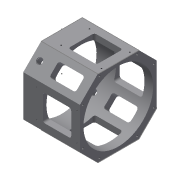
# Autodesk Inventor part: Chamber_wall_NEW_v_4
Saved by Autodesk Inventor 2013 (Build 170138000, 138)
## iProperties
Created: 2012-06-12
Part Number: Chamber_wall_NEW_v_4
Material: Generic
Document SubType Name: Sheet Metal
Designer: Breckenridge2 User
Density: 1 g/cm^3
Sheet Metal Rule: Default
Author: Breckenridge2 User
Autodesk Inventor part; units mm, degrees
ref_plane "YZ Plane" through (0, 0, 0) normal (1, 0, 0) x (0, 1, 0)
ref_plane "XZ Plane" through (0, 0, 0) normal (0, 1, 0) x (-1, 0, 0)
ref_plane "XY Plane" through (0, 0, 0) normal (0, 0, 1) x (1, 0, 0)
sketch "Sketch1" plane through (0, 0, 0) normal (1, 0, 0) x (0, 1, 0)
  point P0 (0, 0)
sketch "Sketch2" plane through (0, 0, 0) normal (1, 0, 0) x (0, 1, 0)
  circle A0 centre (0, 0) radius 101.6
  line L0 (-59.69, 112.014) -> (59.69, 112.014)
  line L1 (59.69, -112.014) -> (-59.69, -112.014)
  line L2 (-59.69, 112.014) -> (59.69, -112.014) construction
  line L3 (59.69, 112.014) -> (-59.69, -112.014) construction
  line L4 (112.014, 59.69) -> (112.014, -59.69)
  line L5 (-112.014, -59.69) -> (-112.014, 59.69)
  line L6 (-112.014, 59.69) -> (112.014, -59.69) construction
  line L7 (112.014, 59.69) -> (-112.014, -59.69) construction
  line L8 (-112.014, 59.69) -> (-59.69, 112.014)
  line L9 (59.69, 112.014) -> (112.014, 59.69)
  line L10 (112.014, -59.69) -> (59.69, -112.014)
  line L11 (-59.69, -112.014) -> (-112.014, -59.69)
  dimension "d1" = 203.2
  dimension "d2" = 119.38
  dimension "d3" = 224.028
  dimension "d4" = 224.028
  dimension "d5" = 119.38
  constraints: 24 end point, 4 midpoint, 2 parallel, 1 centre point, 1 horizontal
  measures "d1" diameter of A0
  measures "d2" distance of L1.start L1.end
  measures "d3" distance of L0.end L1.start
  measures "d4" distance of L4.end L5.start
  measures "d5" distance of L4.start L4.end
extrude "Extrusion1" add sketch "Sketch2" along normal blind 165.1
sketch "Sketch3" plane through (0, 112.014, 59.69) normal (0, 1, 0) x (1, 0, 0)
  line L0 (0, 0) -> (0, 119.38) projected
  line L1 (0, 0) -> (165.1, 0) projected
  line L2 (165.1, 119.38) -> (165.1, 0) projected
  line L3 (0, 119.38) -> (165.1, 119.38) projected
  point P0 (0, 59.69)
sketch "Sketch4" plane through (0, 112.014, 59.69) normal (0, 1, 0) x (1, 0, 0)
  line L0 (133.35, 97.79) -> (63.5, 97.79)
  line L1 (57.15, 91.44) -> (57.15, 27.94)
  line L2 (63.5, 21.59) -> (133.35, 21.59)
  line L3 (139.7, 27.94) -> (139.7, 91.44)
  arc A0 (63.5, 97.79) -> (57.15, 91.44) centre (63.5, 91.44) ccw
  arc A1 (139.7, 91.44) -> (133.35, 97.79) centre (133.35, 91.44) ccw
  arc A2 (133.35, 21.59) -> (139.7, 27.94) centre (133.35, 27.94) ccw
  arc A3 (57.15, 27.94) -> (63.5, 21.59) centre (63.5, 27.94) ccw
  point P0 (0, 59.69)
  point P1 (57.15, 21.59)
  point P2 (57.15, 97.79)
  point P3 (139.7, 21.59)
  dimension "d10" = 82.55
  dimension "d11" = 76.2
  dimension "d12" = 6.35
  constraints: 8 end point, 8 point on circle, 8 tangent, 6 point on line, 4 centre point, 3 equal radius, 2 parallel, 1 horizontal, 1 perpendicular
  measures "d10" distance of point (139.7, 21.59) point (57.15, 21.59)
  measures "d11" distance of point (57.15, 21.59) point (57.15, 97.79)
  measures "d12" radius of A0
extrude "Cut1" cut sketch "Sketch4" against normal up to next
sketch "Sketch5" plane through (0, 112.014, 59.69) normal (0, 1, 0) x (1, 0, 0)
  line L0 (0, 0) -> (0, 119.38) projected
  line L1 (0, 0) -> (165.1, 0) projected
  line L2 (165.1, 119.38) -> (165.1, 0) projected
  line L3 (0, 119.38) -> (165.1, 119.38) projected
  point P0 (0, 59.69)
sketch "Sketch6" plane through (0, -59.69, -112.014) normal (0, 0, -1) x (-1, 0, 0)
  line L0 (-133.35, 97.79) -> (-63.5, 97.79)
  line L1 (-57.15, 91.44) -> (-57.15, 27.94)
  line L2 (-63.5, 21.59) -> (-133.35, 21.59)
  line L3 (-139.7, 27.94) -> (-139.7, 91.44)
  arc A0 (-57.15, 91.44) -> (-63.5, 97.79) centre (-63.5, 91.44) ccw
  arc A1 (-63.5, 21.59) -> (-57.15, 27.94) centre (-63.5, 27.94) ccw
  arc A2 (-133.35, 97.79) -> (-139.7, 91.44) centre (-133.35, 91.44) ccw
  arc A3 (-139.7, 27.94) -> (-133.35, 21.59) centre (-133.35, 27.94) ccw
  point P0 (0, 59.69)
  point P1 (-57.15, 21.59)
  point P2 (-57.15, 97.79)
  point P3 (-139.7, 21.59)
  dimension "d17" = 82.55
  dimension "d18" = 76.2
  dimension "d19" = 6.35
  constraints: 8 end point, 8 point on circle, 8 tangent, 6 point on line, 4 centre point, 3 equal radius, 2 parallel, 1 horizontal, 1 perpendicular
  measures "d17" distance of point (-57.15, 21.59) point (-139.7, 21.59)
  measures "d18" distance of point (-57.15, 97.79) point (-57.15, 21.59)
  measures "d19" radius of A0
extrude "Cut2" cut sketch "Sketch6" against normal up to next
sketch "Sketch7" plane through (0, -112.014, -59.69) normal (0, -1, 0) x (1, 0, 0)
  line L0 (0, 0) -> (0, 119.38) projected
  line L1 (0, 0) -> (165.1, 0) projected
  line L2 (165.1, 119.38) -> (165.1, 0) projected
  line L3 (0, 119.38) -> (165.1, 119.38) projected
  point P0 (0, 59.69)
sketch "Sketch8" plane through (165.1, -59.69, -112.014) normal (0, -0.7071068, -0.7071068) x (-1, 0, 0)
  line L0 (165.1, 0) -> (165.1, -73.9973) projected
  line L1 (165.1, 0) -> (0, 0) projected
  line L2 (0, -73.9973) -> (0, 0) projected
  line L3 (165.1, -73.9973) -> (0, -73.9973) projected
  point P0 (165.1, -36.9987)
sketch "Sketch9" plane through (0, -112.014, -59.69) normal (0, -1, 0) x (1, 0, 0)
  line L0 (133.35, 97.79) -> (63.5, 97.79)
  line L1 (57.15, 91.44) -> (57.15, 27.94)
  line L2 (63.5, 21.59) -> (133.35, 21.59)
  line L3 (139.7, 27.94) -> (139.7, 91.44)
  arc A0 (63.5, 97.79) -> (57.15, 91.44) centre (63.5, 91.44) ccw
  arc A1 (139.7, 91.44) -> (133.35, 97.79) centre (133.35, 91.44) ccw
  arc A2 (133.35, 21.59) -> (139.7, 27.94) centre (133.35, 27.94) ccw
  arc A3 (57.15, 27.94) -> (63.5, 21.59) centre (63.5, 27.94) ccw
  point P0 (0, 59.69)
  point P1 (57.15, 21.59)
  point P2 (57.15, 97.79)
  point P3 (139.7, 21.59)
  dimension "d24" = 82.55
  dimension "d25" = 76.2
  dimension "d26" = 6.35
  constraints: 8 end point, 8 point on circle, 8 tangent, 6 point on line, 4 centre point, 3 equal radius, 2 parallel, 1 horizontal, 1 perpendicular
  measures "d24" distance of point (139.7, 21.59) point (57.15, 21.59)
  measures "d25" distance of point (57.15, 21.59) point (57.15, 97.79)
  measures "d26" radius of A0
extrude "Cut3" cut sketch "Sketch9" against normal up to next
sketch "Sketch10" plane through (0, -59.69, 112.014) normal (0, 0, 1) x (1, 0, 0)
  line L0 (133.35, 97.79) -> (63.5, 97.79)
  line L1 (57.15, 91.44) -> (57.15, 27.94)
  line L2 (63.5, 21.59) -> (133.35, 21.59)
  line L3 (139.7, 27.94) -> (139.7, 91.44)
  arc A0 (63.5, 97.79) -> (57.15, 91.44) centre (63.5, 91.44) ccw
  arc A1 (57.15, 27.94) -> (63.5, 21.59) centre (63.5, 27.94) ccw
  arc A2 (139.7, 91.44) -> (133.35, 97.79) centre (133.35, 91.44) ccw
  arc A3 (133.35, 21.59) -> (139.7, 27.94) centre (133.35, 27.94) ccw
  point P0 (57.15, 21.59)
  point P1 (57.15, 97.79)
  point P2 (139.7, 21.59)
  dimension "d31" = 82.55
  dimension "d32" = 76.2
  constraints: 8 end point, 8 point on circle, 8 tangent, 6 point on line, 4 centre point, 3 equal radius, 2 parallel, 1 horizontal, 1 perpendicular
  measures "d31" distance of point (139.7, 21.59) point (57.15, 21.59)
  measures "d32" distance of point (57.15, 21.59) point (57.15, 97.79)
extrude "Cut4" cut sketch "Sketch10" against normal up to next
sketch "Sketch11" plane through (165.1, -59.69, -112.014) normal (0, -0.7071068, -0.7071068) x (-1, 0, 0)
  line L0 (0, 0) -> (25.4, 0)
  line L1 (25.4, 0) -> (25.4, -17.907)
  line L2 (31.75, -17.907) -> (95.25, -17.907)
  line L3 (101.6, -24.257) -> (101.6, -49.657)
  line L4 (95.25, -56.007) -> (31.75, -56.007)
  line L5 (25.4, -49.657) -> (25.4, -24.257)
  arc A0 (101.6, -24.257) -> (95.25, -17.907) centre (95.25, -24.257) ccw
  arc A1 (95.25, -56.007) -> (101.6, -49.657) centre (95.25, -49.657) ccw
  arc A2 (25.4, -49.657) -> (31.75, -56.007) centre (31.75, -49.657) ccw
  arc A3 (31.75, -17.907) -> (25.4, -24.257) centre (31.75, -24.257) ccw
  point P0 (165.1, -36.9987)
  point P1 (101.6, -56.007)
  point P2 (101.6, -17.907)
  point P3 (25.4, -56.007)
  dimension "d37" = 17.907
  dimension "d38" = 76.2
  dimension "d39" = 38.1
  dimension "d40" = 6.35
  constraints: 12 end point, 8 point on circle, 8 point on line, 8 tangent, 4 centre point, 3 equal radius, 2 horizontal, 2 parallel, 2 perpendicular
  measures "d37" distance of L0.end L1.end
  measures "d38" distance of point (101.6, -56.007) point (25.4, -56.007)
  measures "d39" distance of point (101.6, -17.907) point (101.6, -56.007)
  measures "d40" radius of A0
extrude "Cut5" cut sketch "Sketch11" against normal up to next
sketch "Sketch12" plane through (165.1, -59.69, -112.014) normal (0, -0.7071068, -0.7071068) x (-1, 0, 0)
  line L0 (0, 0) -> (143.51, 0)
  line L1 (143.51, 0) -> (143.51, -36.957)
  line L2 (143.51, -36.957) -> (0, -36.957)
  line L3 (0, -36.957) -> (0, 0)
  circle A0 centre (143.51, -36.957) radius 7.9375
  circle A1 centre (143.51, -36.957) radius 8.6995
  point P0 (165.1, -36.9987)
  dimension "d43" = 143.51
  dimension "d44" = 36.957
  dimension "d45" = 15.875
  dimension "d46" = 17.399
  constraints: 8 end point, 2 centre point, 2 coincident, 2 parallel, 1 horizontal, 1 perpendicular
  measures "d43" distance of L1.end L2.end
  measures "d44" distance of L0.end L1.end
  measures "d45" diameter of A0
  measures "d46" diameter of A1
extrude "Cut6" cut sketch "Sketch12" against normal up to next contours A0 L2 L1 | L1 L2 A0
sketch "Sketch13" plane through (165.1, -59.69, -112.014) normal (0, -0.7071068, -0.7071068) x (-1, 0, 0)
  circle A0 centre (143.51, -36.957) radius 7.9375 projected
  circle A1 centre (143.51, -36.957) radius 8.6995
  point P0 (165.1, -36.9987)
  dimension "d49" = 17.399
  constraints: 1 centre point, 1 coincident
  measures "d49" diameter of A1
extrude "Cut7" cut sketch "Sketch13" against normal blind 2.54
sketch "Sketch14" plane through (165.1, 112.014, -59.69) normal (0, 0.7071068, -0.7071068) x (-1, 0, 0)
  line L0 (31.75, -17.907) -> (95.25, -17.907)
  line L1 (101.6, -24.257) -> (101.6, -49.657)
  line L2 (95.25, -56.007) -> (31.75, -56.007)
  line L3 (25.4, -49.657) -> (25.4, -24.257)
  arc A0 (101.6, -24.257) -> (95.25, -17.907) centre (95.25, -24.257) ccw
  arc A1 (95.25, -56.007) -> (101.6, -49.657) centre (95.25, -49.657) ccw
  arc A2 (25.4, -49.657) -> (31.75, -56.007) centre (31.75, -49.657) ccw
  arc A3 (31.75, -17.907) -> (25.4, -24.257) centre (31.75, -24.257) ccw
  point P0 (165.1, -36.9987)
  point P1 (101.6, -56.007)
  point P2 (101.6, -17.907)
  point P3 (25.4, -56.007)
  dimension "d54" = 76.2
  dimension "d55" = 38.1
  dimension "d56" = 6.35
  constraints: 8 end point, 8 point on circle, 8 tangent, 6 point on line, 4 centre point, 3 equal radius, 2 parallel, 1 horizontal, 1 perpendicular
  measures "d54" distance of point (101.6, -56.007) point (25.4, -56.007)
  measures "d55" distance of point (101.6, -17.907) point (101.6, -56.007)
  measures "d56" radius of A0
extrude "Cut8" cut sketch "Sketch14" against normal up to next
sketch "Sketch15" plane through (165.1, 112.014, -59.69) normal (0, 0.7071068, -0.7071068) x (-1, 0, 0)
  line L0 (0, 0) -> (143.51, 0)
  line L1 (143.51, 0) -> (143.51, -36.957)
  line L2 (143.51, -36.957) -> (0, -36.957)
  line L3 (0, -36.957) -> (0, 0)
  circle A0 centre (143.51, -36.957) radius 7.9375
  point P0 (165.1, -36.9987)
  dimension "d59" = 143.51
  dimension "d60" = 36.957
  dimension "d61" = 15.875
  constraints: 8 end point, 2 parallel, 1 centre point, 1 coincident, 1 horizontal, 1 perpendicular
  measures "d59" distance of L1.end L2.end
  measures "d60" distance of L0.end L1.end
  measures "d61" diameter of A0
extrude "Cut9" cut sketch "Sketch15" against normal up to next contours A0 L2 L1 | L1 L2 A0
sketch "Sketch16" plane through (165.1, 112.014, -59.69) normal (0, 0.7071068, -0.7071068) x (-1, 0, 0)
  circle A0 centre (143.51, -36.957) radius 7.9375 projected
  circle A1 centre (143.51, -36.957) radius 8.6995
  point P0 (165.1, -36.9987)
  dimension "d64" = 17.399
  constraints: 1 centre point, 1 coincident
  measures "d64" diameter of A1
extrude "Cut10" cut sketch "Sketch16" against normal blind 2.54
sketch "Sketch17" plane through (0, 59.69, 112.014) normal (0, 0.7071068, 0.7071068) x (1, 0, 0)
  line L0 (133.35, 56.0903) -> (69.85, 56.0903)
  line L1 (63.5, 49.7403) -> (63.5, 24.3403)
  line L2 (69.85, 17.9903) -> (133.35, 17.9903)
  line L3 (139.7, 24.3403) -> (139.7, 49.7403)
  arc A0 (69.85, 56.0903) -> (63.5, 49.7403) centre (69.85, 49.7403) ccw
  arc A1 (139.7, 49.7403) -> (133.35, 56.0903) centre (133.35, 49.7403) ccw
  arc A2 (133.35, 17.9903) -> (139.7, 24.3403) centre (133.35, 24.3403) ccw
  arc A3 (63.5, 24.3403) -> (69.85, 17.9903) centre (69.85, 24.3403) ccw
  point P0 (0, 36.9987)
  point P1 (63.5, 17.9903)
  point P2 (63.5, 56.0903)
  point P3 (139.7, 17.9903)
  dimension "d69" = 76.2
  dimension "d70" = 38.1
  dimension "d71" = 6.35
  constraints: 8 end point, 8 point on circle, 8 tangent, 6 point on line, 4 centre point, 3 equal radius, 2 parallel, 1 horizontal, 1 perpendicular
  measures "d69" distance of point (139.7, 17.99) point (63.5, 17.99)
  measures "d70" distance of point (63.5, 17.99) point (63.5, 56.09)
  measures "d71" radius of A0
extrude "Cut11" cut sketch "Sketch17" against normal up to next
sketch "Sketch18" plane through (0, 59.69, 112.014) normal (0, 0.7071068, 0.7071068) x (1, 0, 0)
  line L0 (165.1, 0) -> (21.59, 0)
  line L1 (21.59, 0) -> (21.59, 36.957)
  line L2 (21.59, 36.957) -> (165.1, 36.957)
  line L3 (165.1, 36.957) -> (165.1, 0)
  circle A0 centre (21.59, 36.957) radius 7.9375
  point P0 (0, 36.9987)
  dimension "d74" = 143.51
  dimension "d75" = 36.957
  dimension "d76" = 15.875
  constraints: 8 end point, 2 parallel, 1 centre point, 1 coincident, 1 horizontal, 1 perpendicular
  measures "d74" distance of L1.end L2.end
  measures "d75" distance of L0.end L1.end
  measures "d76" diameter of A0
extrude "Cut12" cut sketch "Sketch18" against normal up to next contours A0 L2 L1 | L1 L2 A0
sketch "Sketch19" plane through (0, 59.69, 112.014) normal (0, 0.7071068, 0.7071068) x (1, 0, 0)
  circle A0 centre (21.59, 36.957) radius 7.9375 projected
  circle A1 centre (21.59, 36.957) radius 8.6995
  point P0 (0, 36.9987)
  dimension "d79" = 17.399
  constraints: 1 centre point, 1 coincident
  measures "d79" diameter of A1
extrude "Cut13" cut sketch "Sketch19" against normal blind 2.54
sketch "Sketch20" plane through (0, -112.014, 59.69) normal (0, -0.7071068, 0.7071068) x (1, 0, 0)
  line L0 (133.35, 56.0903) -> (69.85, 56.0903)
  line L1 (63.5, 49.7403) -> (63.5, 24.3403)
  line L2 (69.85, 17.9903) -> (133.35, 17.9903)
  line L3 (139.7, 24.3403) -> (139.7, 49.7403)
  arc A0 (69.85, 56.0903) -> (63.5, 49.7403) centre (69.85, 49.7403) ccw
  arc A1 (139.7, 49.7403) -> (133.35, 56.0903) centre (133.35, 49.7403) ccw
  arc A2 (133.35, 17.9903) -> (139.7, 24.3403) centre (133.35, 24.3403) ccw
  arc A3 (63.5, 24.3403) -> (69.85, 17.9903) centre (69.85, 24.3403) ccw
  point P0 (0, 36.9987)
  point P1 (63.5, 17.9903)
  point P2 (63.5, 56.0903)
  point P3 (139.7, 17.9903)
  dimension "d84" = 76.2
  dimension "d85" = 38.1
  dimension "d86" = 6.35
  constraints: 8 end point, 8 point on circle, 8 tangent, 6 point on line, 4 centre point, 3 equal radius, 2 parallel, 1 horizontal, 1 perpendicular
  measures "d84" distance of point (139.7, 17.99) point (63.5, 17.99)
  measures "d85" distance of point (63.5, 17.99) point (63.5, 56.09)
  measures "d86" radius of A0
extrude "Cut14" cut sketch "Sketch20" against normal up to next
sketch "Sketch21" plane through (0, -112.014, 59.69) normal (0, -0.7071068, 0.7071068) x (1, 0, 0)
  line L0 (165.1, 0) -> (21.59, 0)
  line L1 (21.59, 0) -> (21.59, 36.957)
  line L2 (21.59, 36.957) -> (165.1, 36.957)
  line L3 (165.1, 36.957) -> (165.1, 0)
  circle A0 centre (21.59, 36.957) radius 7.9375
  point P0 (0, 36.9987)
  dimension "d89" = 143.51
  dimension "d90" = 36.957
  dimension "d91" = 15.875
  constraints: 8 end point, 2 parallel, 1 centre point, 1 coincident, 1 horizontal, 1 perpendicular
  measures "d89" distance of L1.end L2.end
  measures "d90" distance of L0.end L1.end
  measures "d91" diameter of A0
extrude "Cut15" cut sketch "Sketch21" against normal up to next contours A0 L2 L1 | L1 L2 A0
sketch "Sketch22" plane through (0, -112.014, 59.69) normal (0, -0.7071068, 0.7071068) x (1, 0, 0)
  circle A0 centre (21.59, 36.957) radius 7.9375 projected
  circle A1 centre (21.59, 36.957) radius 8.6995
  point P0 (0, 36.9987)
  dimension "d94" = 17.399
  constraints: 1 centre point, 1 coincident
  measures "d94" diameter of A1
extrude "Cut16" cut sketch "Sketch22" against normal blind 2.54
sketch "Sketch23" plane through (165.1, 0, 0) normal (1, 0, 0) x (0, 0, -1)
  point P0 (-103.1134, 54.9471)
  point P1 (-54.9471, 103.1134)
  point P2 (54.9471, 103.1134)
  point P3 (103.1134, 54.9471)
  point P4 (103.1134, -54.9471)
  point P5 (54.9471, -103.1134)
  point P6 (-54.9471, -103.1134)
  point P7 (-103.1134, -54.9471)
hole "Hole1" at (165.1, 54.9471, 103.1134) at (165.1, 103.1134, 54.9471) at (165.1, 103.1134, -54.9471) at (165.1, 54.9471, -103.1134) at (165.1, -54.9471, -103.1134) at (165.1, -103.1134, -54.9471) at (165.1, -103.1134, 54.9471) at (165.1, -54.9471, 103.1134) direction (-1, 0, 0) diameter 4.9784 depth 18.415 tip angle 118 thread size "1/4-20 UNC" class "2B" standard "ANSI Unified Screw Threads"
sketch "Sketch24" plane through (0, 0, 0) normal (-1, 0, 0) x (0, 0, 1)
  point P0 (-103.1134, 54.9471)
  point P1 (-54.9471, 103.1134)
  point P2 (54.9471, 103.1134)
  point P3 (103.1134, 54.9471)
  point P4 (103.1134, -54.9471)
  point P5 (54.9471, -103.1134)
  point P6 (-54.9471, -103.1134)
  point P7 (-103.1134, -54.9471)
hole "Hole2" at (0, 54.9471, -103.1134) at (0, 103.1134, -54.9471) at (0, 103.1134, 54.9471) at (0, 54.9471, 103.1134) at (0, -54.9471, 103.1134) at (0, -103.1134, 54.9471) at (0, -103.1134, -54.9471) at (0, -54.9471, -103.1134) direction (1, 0, 0) diameter 4.9784 depth 18.415 tip angle 118 thread size "1/4-20 UNC" class "2B" standard "ANSI Unified Screw Threads"
sketch "Sketch25" plane through (0, -59.69, 112.014) normal (0, 0, 1) x (1, 0, 0)
  point P0 (0, 59.69)
  point P1 (157.226, 100.965)
  point P2 (39.624, 100.965)
  point P3 (39.624, 18.415)
  point P4 (157.226, 18.415)
hole "Hole3" at (39.624, 41.275, 112.014) at (157.226, 41.275, 112.014) at (39.624, -41.275, 112.014) at (157.226, -41.275, 112.014) direction (0, 0, -1) diameter 3.9624 depth 13.97 tip angle 118 thread size "10-32 UNF" class "2B" standard "ANSI Unified Screw Threads"
sketch "Sketch26" plane through (0, 112.014, 59.69) normal (0, 1, 0) x (1, 0, 0)
  point P0 (0, 59.69)
  point P1 (157.226, 100.965)
  point P2 (39.624, 100.965)
  point P3 (39.624, 18.415)
  point P4 (157.226, 18.415)
  point P5 (157.226, 100.965)
  constraints: 1 coincident
hole "Hole4" at (39.624, 112.014, 41.275) at (39.624, 112.014, -41.275) at (157.226, 112.014, -41.275) at (157.226, 112.014, 41.275) direction (0, -1, 0) diameter 3.9624 depth 13.97 tip angle 118 thread size "10-32 UNF" class "2B" standard "ANSI Unified Screw Threads"
sketch "Sketch27" plane through (0, -112.014, -59.69) normal (0, -1, 0) x (1, 0, 0)
  point P0 (0, 59.69)
  point P1 (157.226, 100.965)
  point P2 (39.624, 100.965)
  point P3 (39.624, 18.415)
  point P4 (157.226, 18.415)
hole "Hole5" at (157.226, -112.014, 41.275) at (157.226, -112.014, -41.275) at (39.624, -112.014, 41.275) at (39.624, -112.014, -41.275) direction (0, 1, 0) diameter 3.9624 depth 13.97 tip angle 118 thread size "10-32 UNF" class "2B" standard "ANSI Unified Screw Threads"
sketch "Sketch28" plane through (0, -59.69, -112.014) normal (0, 0, -1) x (-1, 0, 0)
  point P0 (0, 59.69)
  point P1 (-157.226, 100.965)
  point P2 (-157.226, 18.415)
  point P3 (-39.624, 18.415)
  point P4 (-39.624, 100.965)
hole "Hole6" at (157.226, -41.275, -112.014) at (157.226, 41.275, -112.014) at (39.624, 41.275, -112.014) at (39.624, -41.275, -112.014) direction (0, 0, 1) diameter 3.9624 depth 13.97 tip angle 118 thread size "10-32 UNF" class "2B" standard "ANSI Unified Screw Threads"
equation "\"d13\" = Thickness"
equation "\"d20\" = Thickness"
equation "\"d27\" = Thickness"
equation "\"d34\" = Thickness"
equation "\"d41\" = Thickness"
equation "\"d47\" = Thickness"
equation "\"d57\" = Thickness"
equation "\"d62\" = Thickness"
equation "\"d72\" = Thickness"
equation "\"d77\" = Thickness"
equation "\"d87\" = Thickness"
equation "\"d92\" = Thickness"
equation "\"BendRadius\" = Thickness"
equation "\"BendReliefWidth\" = Thickness"
equation "\"BendReliefDepth\" = 0.5 * Thickness"
equation "\"CornerReliefSize\" = 4 * Thickness"
equation "\"MinimumRemnant\" = 2 * Thickness"
equation "\"TransitionRadius\" = BendRadius"
equation "\"JacobiRadiusSize\" = BendRadius"
equation "\"GapSize\" = Thickness"
equation "\"Thickness\" = 3.048"
body "Solid1"
